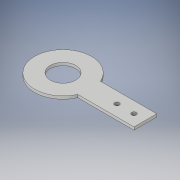
# Autodesk Inventor part: wheel tip
Saved by Autodesk Inventor 2018 (Build 220112000, 112)
## iProperties
Created: 2019-01-23
Part Number: wheel tip
Material: Generic
Document SubType Name: Modeling
Designer: s-2513225
Density: 1 g/cm^3
Appearance: Default
Author: s-2513225
Autodesk Inventor part; units mm, degrees
ref_plane "YZ Plane" through (0, 0, 0) normal (1, 0, 0) x (0, 1, 0)
ref_plane "XZ Plane" through (0, 0, 0) normal (0, 1, 0) x (-1, 0, 0)
ref_plane "XY Plane" through (0, 0, 0) normal (0, 0, 1) x (1, 0, 0)
sketch "Sketch1" plane through (0, 0, 0) normal (0, 1, 0) x (-1, 0, 0)
  line L0 (0, 0) -> (0, -12.7)
  line L1 (0, -12.7) -> (50.8, -12.7)
  line L2 (0, 12.7) -> (50.8, 12.7)
  line L3 (50.8, -12.7) -> (50.8, 0) construction
  line L4 (50.8, 0) -> (79.375, 0) construction
  circle A0 centre (79.375, 0) radius 14.2875
  arc A1 (50.2756, -12.7) -> (50.2756, 12.7) centre (79.375, 0) ccw
  line L5 (0, 0) -> (19.05, 0) construction
  circle A2 centre (19.05, 0) radius 2.5797
  circle A3 centre (0, 0) radius 2.5797
  line L6 (0, -12.7) -> (-12.7, -12.7)
  line L7 (-12.7, -12.7) -> (-12.7, 12.7)
  line L8 (-12.7, 12.7) -> (0, 12.7)
  line L9 (-12.7, 0) -> (0, 0) construction
  dimension "d1" = 50.8
  dimension "d2" = 28.575
  dimension "d3" = 28.575
  dimension "d4" = 63.5
  dimension "d6" = 19.05
  dimension "d7" = 5.1594
  dimension "d8" = 5.1594
  dimension "d11" = 12.7
  dimension "d14" = 12.7
  constraints: 20 end point, 4 centre point, 4 coincident, 4 perpendicular, 2 horizontal, 2 point on circle, 2 point on line, 2 vertical, 1 midpoint
  measures "d1" distance of L0.end L1.end
  measures "d2" distance of L3.end L4.end
  measures "d3" diameter of A0
  measures "d4" diameter of A1
  measures "d6" distance of L5.start L5.end
  measures "d7" diameter of A2
  measures "d8" diameter of A3
  measures "d11" distance of L0.end L6.end
  measures "d14" distance of L9.start L0.start
extrude "Extrusion1" add sketch "Sketch1" along normal blind 3.175
body "Solid1"
